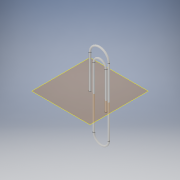
# Autodesk Inventor part: Paper Clip
Saved by Autodesk Inventor 2017 (Build 210142000, 142)
## iProperties
Created: 2020-02-06
Part Number: Paper Clip
Material: Generic
Document SubType Name: Modeling
Designer: 10042265
Density: 1 g/cm^3
Appearance: Default
Author: 10042265
Autodesk Inventor part; units mm, degrees
ref_plane "YZ Plane" through (0, 0, 0) normal (1, 0, 0) x (0, 1, 0)
ref_plane "XZ Plane" through (0, 0, 0) normal (0, 1, 0) x (-1, 0, 0)
ref_plane "XY Plane" through (0, 0, 0) normal (0, 0, 1) x (1, 0, 0)
sketch "Sketch6" plane through (0, 0, 0) normal (0, 0, 1) x (1, 0, 0)
  line L0 (0, 0) -> (0, 12.7)
  arc A0 (7.112, 12.7) -> (0, 12.7) centre (3.556, 12.7) ccw
  line L1 (7.112, 12.7) -> (7.112, -12.7)
  arc A1 (1.4732, -12.7) -> (7.112, -12.7) centre (4.2926, -12.7) ccw
  line L2 (1.4732, -12.7) -> (1.4732, 10.16)
  arc A2 (6.0452, 10.16) -> (1.4732, 10.16) centre (3.7592, 10.16) ccw
  line L3 (6.0452, 10.16) -> (6.0452, -3.81)
  dimension "d1" = 12.7
  dimension "d2" = 25.4
  dimension "d3" = 5.6388
  dimension "d4" = 4.572
  dimension "d5" = 13.97
  dimension "d6" = 22.86
  dimension "d7" = 3.556
  constraints: 8 end point, 6 point on circle, 6 tangent, 4 vertical, 3 centre point
  measures "d1" distance of L0.start L0.end
  measures "d2" distance of L1.start L1.end
  measures "d3" diameter of A1
  measures "d4" diameter of A2
  measures "d5" distance of L3.start L3.end
  measures "d6" distance of L2.start L2.end
  measures "d7" radius of A0
ref_plane "Work Plane1" through (0, 0, 0) normal (0, 1, 0) x (-1, 0, 0)
sketch "Sketch7" plane through (0, 0, 0) normal (0, 1, 0) x (-1, 0, 0)
  circle A0 centre (0, 0) radius 0.3175
  dimension "d8" = 0.635
  constraints: 1 centre point, 1 coincident
  measures "d8" diameter of A0
sweep "Sweep1" add profiles "Sketch7" path "Sketch6"
body "Solid1"
